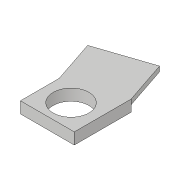
# Autodesk Inventor part: Lidar Sensor CAse Piece 1
Saved by Autodesk Inventor 2018.3 (Build 223284000, 284)
## iProperties
Created: 2019-02-15
Part Number: Lidar Sensor CAse Piece 1
Material: Generic
Document SubType Name: Modeling
Designer: aye06091
Mass: 5.1775 g
Surface Area: 32.7073 cm^2
Volume: 5.1775 cm^3
Density: 1 g/cm^3
Appearance: Default
Author: aye06091
Autodesk Inventor part; units mm, degrees
ref_plane "YZ Plane" through (0, 0, 0) normal (1, 0, 0) x (0, 1, 0)
ref_plane "XZ Plane" through (0, 0, 0) normal (0, 1, 0) x (-1, 0, 0)
ref_plane "XY Plane" through (0, 0, 0) normal (0, 0, 1) x (1, 0, 0)
sketch "Sketch1" plane through (0, 0, 0) normal (0, 1, 0) x (-1, 0, 0)
  line L0 (-8.0312, -19.6194) -> (-8.0312, -0.5694)
  line L1 (-8.0312, -0.5694) -> (-34.5277, -0.5694)
  line L2 (-34.5277, -0.5694) -> (-34.5277, -28.5056)
  line L3 (18.6455, 5.0782) -> (18.6456, 5.0782)
  line L4 (-1.974, -37.6808) -> (-8.0312, -19.6194)
  line L5 (-34.5277, -28.5056) -> (-27.4611, -49.5771)
  line L6 (-1.974, -37.6808) -> (-0.9645, -40.691)
  line L7 (-27.4611, -49.5771) -> (-0.9645, -40.691)
  circle A0 centre (-21.2794, -12.2217) radius 8.7948
  line L8 (-8.0312, -0.5694) -> (-8.0312, -19.6194)
  line L9 (-8.0312, -19.6194) -> (-0.9645, -40.691)
  line L10 (-0.9645, -40.691) -> (-27.4611, -49.5771)
  line L11 (-27.4611, -49.5771) -> (-34.5277, -28.5056)
  line L12 (-34.5277, -28.5056) -> (-34.5277, -0.5694)
  line L13 (-34.5277, -0.5694) -> (-8.0312, -0.5694)
  dimension "d0" = 19.05
  dimension "d1" = 22.225
  dimension "d2" = 27.9469
  dimension "d3" = 26.4965
  dimension "d4" = 17.5895
  dimension "d18" = 13.2483
  dimension "d20" = 161.46
  dimension "d26" = 11.6523
  constraints: 28 end point, 3 perpendicular, 2 parallel, 1 centre point, 1 collinear, 1 vertical
  measures "d0" distance of L0.start L0.end
  measures "d1" distance of L4.end L6.end
  measures "d2" distance of L5.end L7.end
  measures "d3" distance of L0.end L1.end
  measures "d4" diameter of A0
  measures "d18" distance from line of A0.centre L2
  measures "d20" angle of L4 L0
  measures "d26" distance from line of L1 A0.centre
extrude "Extrusion1" add sketch "Sketch1" along normal blind 5.6134
sketch "Sketch2" plane through (0, 0, 0) normal (0, -1, 0) x (1, 0, 0)
  line L0 (27.4611, -49.5771) -> (0.9645, -40.691) projected
  line L1 (28.4833, -26.4785) -> (28.4832, -26.4784)
  line L2 (8.0312, -19.6194) -> (7.0701, -22.4851)
  line L3 (27.461, -49.5772) -> (24.8, -48.6848)
  line L4 (27.4611, -49.5771) -> (24.8, -48.6846)
  line L5 (34.5277, -28.5056) -> (27.4611, -49.5771) projected
  line L6 (34.5277, -0.5694) -> (34.5277, -28.5056) projected
  line L7 (30.9057, -30.4788) -> (24.8, -48.6846)
  line L8 (24.8, -48.6846) -> (27.4611, -49.5771)
  line L9 (27.4611, -49.5771) -> (34.5277, -28.5056)
  line L10 (0.9645, -40.691) -> (8.0312, -19.6194) projected
  line L11 (34.5277, -0.5694) -> (34.5277, -28.5056) projected
  line L12 (8.0312, -19.6194) -> (34.5277, -28.5056)
  line L13 (8.0312, -19.6194) -> (7.0701, -22.4852)
  line L14 (7.0701, -22.4852) -> (30.9057, -30.4788)
  line L15 (33.5667, -31.3712) -> (34.5278, -28.5055)
  line L16 (34.5278, -28.5055) -> (8.0312, -19.6194)
  point P0 (0, 0)
  point P1 (34.5277, -28.5056)
  dimension "d24" = 2.8067
  dimension "d27" = 3.0226
  constraints: 24 end point, 5 point on line, 3 parallel, 3 perpendicular, 1 collinear
  measures "d24" distance between parallel lines of L7 L9
  measures "d27" distance between parallel lines of L16 L14
extrude "Extrusion2" cut sketch "Sketch2" against normal blind 3.175 contours L0 L7 L14 L2 L12 L5
body "Solid1"
